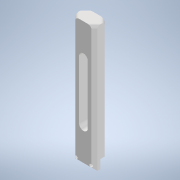
# Autodesk Inventor part: pen_2
Saved by Autodesk Inventor 2020 (Build 240168000, 168)
## iProperties
Created: 2019-11-04
Part Number: pen_2
Material: Generic
Document SubType Name: Modeling
Designer: psrob
Density: 1 g/cm^3
Appearance: Default
Author: psrob
Autodesk Inventor part; units mm, degrees
ref_plane "YZ Plane" through (0, 0, 0) normal (1, 0, 0) x (0, 1, 0)
ref_plane "XZ Plane" through (0, 0, 0) normal (0, 1, 0) x (-1, 0, 0)
ref_plane "XY Plane" through (0, 0, 0) normal (0, 0, 1) x (1, 0, 0)
sketch "Sketch1" plane through (0, 0, 0) normal (0, 0, 1) x (1, 0, 0)
  spline S0 degree 3 poles (5, 2.8134) (4.7282, 2.7718) (4.4577, 2.7171) (3.9725, 2.5829) (3.7572, 2.5096) (3.2649, 2.2994) (2.9924, 2.1483) (2.5895, 1.8431) (2.4453, 1.712) (2.3168, 1.5682) (2.1311, 1.3604) (1.976, 1.1232) (1.7525, 0.5925) (1.6905, 0.2977) (1.6905, 0) knots 0 0 0 0 0.174284 0.174284 0.317468 0.317468 0.513399 0.513399 0.635856 0.635856 0.635856 0.812785 0.812785 1 1 1 1
  line L0 (5, 2.8134) -> (5, 10)
  line L1 (0, 10) -> (5, 10)
  line L2 (0, 2.607) -> (0, 10)
  spline S1 degree 3 poles (1.5054, -1.0718) (1.0443, -0.6134) (0.6771, -0.0703) (0.2854, 0.8445) (0.1821, 1.1739) (0.0367, 1.8715) (0, 2.2339) (0, 2.607) knots 0 0 0 0 0.47732 0.47732 0.730106 0.730106 1 1 1 1
  spline S2 degree 3 poles (1.6905, -1.2645) (1.6303, -1.1989) (1.5686, -1.1346) (1.5054, -1.0718) knots 0 0 0 0 1 1 1 1
  line L3 (1.6905, 0) -> (1.6905, -1.2645)
  circle A0 centre (2.5, 7) radius 1
  circle A1 centre (12.5, 7) radius 1
  spline S3 degree 3 poles (13.3095, 0) (13.3095, 0.2448) (13.2668, 0.4921) (13.0809, 1.0308) (12.9041, 1.3201) (12.6871, 1.5639) (12.5591, 1.7077) (12.4154, 1.8388) (12.0138, 2.1444) (11.7421, 2.2958) (11.2512, 2.5065) (11.0368, 2.5799) (10.5491, 2.7158) (10.2752, 2.7712) (10, 2.8134) knots 0 0 0 0 0.154789 0.154789 0.362213 0.362213 0.362213 0.4846 0.4846 0.68042 0.68042 0.823311 0.823311 1 1 1 1
  line L4 (13.3095, -1.2645) -> (13.3095, 0)
  spline S4 degree 3 poles (13.3095, -1.2645) (13.3697, -1.1989) (13.4314, -1.1346) (13.4946, -1.0718) knots 0 0 0 0 1 1 1 1
  spline S5 degree 3 poles (15, 2.607) (15, 2.4473) (14.9933, 2.2901) (14.9258, 1.5152) (14.7659, 0.9156) (14.2513, -0.1742) (13.9111, -0.6578) (13.4946, -1.0718) knots 0 0 0 0 0.115959 0.115959 0.56908 0.56908 1 1 1 1
  line L5 (15, 2.607) -> (15, 10)
  line L6 (10, 10) -> (15, 10)
  line L7 (10, 10) -> (10, 2.8134)
  line L8 (0, 10) -> (15, 10)
  line L9 (15, 10) -> (15, 4)
  line L10 (15, 4) -> (0, 4)
  line L11 (0, 4) -> (0, 10)
  point P0 (0, 0)
  dimension "d0" = 15
  dimension "d1" = 6
  constraints: 8 end point, 2 parallel, 1 horizontal, 1 perpendicular
  measures "d0" distance of L9.end L10.end
  measures "d1" distance of L8.end L9.end
extrude "Extrusion1" add sketch "Sketch1" along normal blind 4 contours L10 L2 L1 L0 | L0 L8 L7 L10 | L7 L6 L5 L10
sketch "Sketch2" plane through (0, 10, 0) normal (0, 1, 0) x (1, 0, 0)
  line L0 (15, 0) -> (0, 0) projected
  line L1 (0, 0) -> (0, -4) projected
  line L2 (15, -4) -> (0, -4) projected
  line L3 (15, 0) -> (15, -4) projected
  line L4 (15, -4) -> (0, -4) projected
  line L5 (0, -4) -> (15, -4)
  line L6 (15, -4) -> (15, 5)
  line L7 (15, 5) -> (0, 5)
  line L8 (0, 5) -> (0, -4)
  dimension "d4" = 15
  dimension "d5" = 9
  constraints: 8 end point, 2 parallel, 1 horizontal, 1 perpendicular
  measures "d4" distance of L7.end L6.end
  measures "d5" distance of L6.end L5.end
extrude "Extrusion2" add sketch "Sketch2" along normal blind 80
sketch "Sketch3" plane through (15, 10, -5) normal (0, 0, -1) x (-1, 0, 0)
  line L0 (0, 0) -> (15, 0) projected
  line L1 (15, 0) -> (15, 80) projected
  line L2 (0, 80) -> (15, 80) projected
  line L3 (0, 0) -> (0, 80) projected
  line L4 (7.5, 80) -> (7.5, 38)
  line L5 (7.5, 18) -> (7.5, 58) construction
  line L6 (10.5, 18) -> (10.5, 58)
  line L7 (4.5, 58) -> (4.5, 18)
  arc A0 (4.5, 18) -> (10.5, 18) centre (7.5, 18) ccw
  arc A1 (10.5, 58) -> (4.5, 58) centre (7.5, 58) ccw
  point P0 (15, -10)
  dimension "d8" = 42
  dimension "d9" = 20
  dimension "d10" = 6
  constraints: 10 end point, 4 point on circle, 4 tangent, 2 centre point, 2 midpoint, 1 parallel, 1 point on line, 1 vertical
  measures "d8" distance of L4.start L4.end
  measures "d9" distance of L4.end L5.end
  measures "d10" diameter of A1
extrude "Extrusion3" cut sketch "Sketch3" against normal blind 80 contours A0 L7 A1 L6
chamfer "Chamfer1" distance 2 angle 45 4 edges at (15, 47, 4) (15, 50, -5) (0, 50, -5) (0, 47, 4)
chamfer "Chamfer2" distance 2 angle 45 1 edges at (7.5, 4, 4)
fillet "Fillet1" radius 2 4 edges at (1, 90, -4) (14, 90, -4) (14, 90, 3) (1, 90, 3)
body "Solid1"
